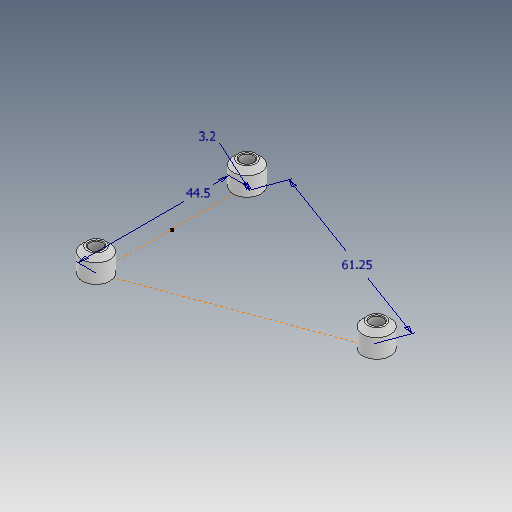
# Autodesk Inventor part: db-25_standoffs_plate
Saved by Autodesk Inventor 2025.1 (Build 291241000, 241)
## iProperties
Created: 2026-06-20
Part Number: db-25_standoffs_plate
Material: Generic
Document SubType Name: Modeling
Designer: Aiden
Density: 1 g/cm^3
Appearance: Default
Author: Aiden
Autodesk Inventor part; units mm, degrees
ref_plane "YZ Plane" through (0, 0, 0) normal (1, 0, 0) x (0, 1, 0)
ref_plane "XZ Plane" through (0, 0, 0) normal (0, 1, 0) x (-1, 0, 0)
ref_plane "XY Plane" through (0, 0, 0) normal (0, 0, 1) x (1, 0, 0)
sketch "Sketch1" plane through (0, 0, 0) normal (0, 1, 0) x (-1, 0, 0)
  circle A0 centre (42.9488, 7.9638) radius 1.6 construction
  circle A1 centre (-17.5388, 30.2138) radius 1.6 construction
  circle A2 centre (42.9488, 52.4638) radius 1.6 construction
  line L0 (42.9488, 7.9638) -> (42.9488, 52.4638) construction
  line L1 (41.4471, 51.9114) -> (-16.0371, 30.7661) construction
  point P0 (42.9488, 30.2138)
  dimension "d0" = 3.2
  dimension "d22" = 44.5
  dimension "d23" = 61.25
  constraints: 4 end point, 1 centre point, 1 horizontal alignment, 1 midpoint, 1 vertical, 1 vertical alignment, 10 other
  measures "d0" diameter of A0
  measures "d22" distance of L0.start L0.end
sketch "Sketch2" plane through (0, 0, 0) normal (0, 1, 0) x (-1, 0, 0)
  circle A0 centre (42.9488, 7.9638) radius 1.6 construction
  circle A1 centre (-17.5388, 30.2138) radius 1.6 construction
  circle A2 centre (42.9488, 52.4638) radius 1.6 construction
  circle A3 centre (42.9488, 7.9638) radius 3.1
  circle A4 centre (-17.5388, 30.2138) radius 3.1
  circle A5 centre (42.9488, 52.4638) radius 3.1
  point P0 (0, 0)
  dimension "d6" = 1.5
  constraints: 3 centre point, 3 coincident, 2 equal radius
  measures "d6" radial gap between concentric circles of A0 A3
extrude "Extrusion1" add sketch "Sketch2" along normal blind 7
sketch "Sketch3" plane through (-42.9488, 7, 7.9638) normal (0, 1, 0) x (1, 0, 0)
  circle A0 centre (0, 0) radius 3.1 projected
  circle A1 centre (60.4875, -22.25) radius 3.1 projected
  circle A2 centre (0, -44.5) radius 3.1 projected
  point P0 (42.9488, 7.9638)
  point P1 (81.2288, -33.1404)
  point P2 (81.2288, -33.1404)
  constraints: 4 coincident
hole "Hole1" at (-42.9488, 7, 7.9638) at (17.5388, 7, 30.2138) at (38.2801, 7, 41.1042) at (-42.9488, 7, 52.4638) direction (0, -1, 0) diameter 3.75 end through all
chamfer "Chamfer1" distance 0.2 angle 45 3 edges at (-42.9488, 7, 6.0888) (17.5388, 7, 28.3388) (-42.9488, 7, 50.5888)
thicken "Thicken1" operation add thickness 1 both sides no extend neighbours no toward (-0.9870503, 0, -0.1604113) faces at (-46.0086, 4.6667, 7.4665)
thicken "Thicken2" operation add thickness 1 both sides no extend neighbours no toward (-0.9870503, 0, -0.1604113) faces at (-46.0086, 4.6667, 51.9665)
thicken "Thicken3" operation add thickness 1 both sides no extend neighbours no toward (-0.9870503, 0, -0.1604113) faces at (14.4789, 4.6667, 29.7165)
chamfer "Chamfer2" distance 1.5 angle 45 3 edges at (-38.8488, 7, 7.9638) (-38.8488, 7, 52.4638) (21.6388, 7, 30.2138)
body "Solid1"
